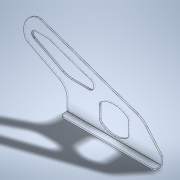
# Autodesk Inventor part: 0 零件
Saved by Autodesk Inventor 2020 (Build 240168000, 168)
## iProperties
Created: 2020-11-03
Part Number: 0 零件
Material: 不鏽鋼
Document SubType Name: Sheet Metal
Designer: p2013
Density: 8 g/cm^3
Appearance: 半拋光
Flat Pattern Width: 10.0917 cm
Flat Pattern Length: 19 cm
Flat Pattern Area: 191.742 cm^2
Sheet Metal Rule: 預設 mm (_M)
Sheet Metal Width: 100.92 mm
Sheet Metal Length: 190.00 mm
Sheet Metal Area: 19174.16 mm^2
Author: p2013
Autodesk Inventor part; units mm, degrees
ref_plane "YZ Plane" through (0, 0, 0) normal (1, 0, 0) x (0, 1, 0)
ref_plane "XZ Plane" through (0, 0, 0) normal (0, 1, 0) x (-1, 0, 0)
ref_plane "XY Plane" through (0, 0, 0) normal (0, 0, 1) x (1, 0, 0)
sketch "草圖1" plane through (0, 0, 0) normal (0, 0, 1) x (1, 0, 0)
  line L0 (0, 0) -> (-40.5681, 0) construction
  line L1 (0, 0) -> (0, 42.2738) construction
  line L2 (-65, 18.7) -> (-19.3972, 18.7) construction
  line L3 (65, 18.7) -> (65, 3.5)
  line L4 (61.5, 0) -> (-61.5, 0)
  line L5 (-65, 3.5) -> (-65, 18.7)
  line L6 (-85.1195, 8.7) -> (78.7394, 8.7)
  arc A0 (-65, 3.5) -> (-61.5, 0) centre (-61.5, 3.5) ccw
  arc A1 (61.5, 0) -> (65, 3.5) centre (61.5, 3.5) ccw
  arc A2 (-18, 17.0607) -> (18, 17.0607) centre (0, 41.0607) ccw
  line L7 (-20, 18.7) -> (20, 18.7) construction
  line L8 (19.3972, 18.7) -> (65, 18.7) construction
  line L9 (-65, 18.7) -> (-65, 23.7)
  line L10 (-75.8518, 41.4851) -> (-119.064, 63.7122)
  line L11 (-101.9165, 99.0537) -> (30.9171, 52.7442)
  line L12 (44.0225, 43.7) -> (65, 18.7)
  arc A3 (44.0225, 43.7) -> (30.9171, 52.7442) centre (21.0412, 24.4164) ccw
  arc A4 (-65, 23.7) -> (-75.8518, 41.4851) centre (-85, 23.7) ccw
  arc A5 (-108.162, 99.165) -> (-124.1228, 69.9202) centre (-101.1042, 76.3353) ccw
  line L13 (-104.5691, 99.9785) -> (-122.3532, 65.4041) construction
  line L14 (-92.566, 80.8091) -> (-108.8509, 80.8091)
  arc A6 (-89.2737, 80.2516) -> (-92.566, 80.8091) centre (-92.566, 70.8091) ccw
  line L15 (-32.7123, 60.5304) -> (-89.2737, 80.2516)
  arc A7 (-108.8509, 80.8091) -> (-110.452, 74.1968) centre (-108.8509, 77.3091) ccw
  line L16 (-110.452, 74.1968) -> (-70.3705, 53.5781)
  arc A8 (-70.3705, 53.5781) -> (-58.9345, 50.8091) centre (-58.9345, 75.8091) ccw
  line L17 (-58.9345, 50.8091) -> (-34.3585, 50.8091)
  arc A9 (-34.3585, 50.8091) -> (-32.7123, 60.5304) centre (-34.3585, 55.8091) ccw
  arc A10 (-88.7798, 81.668) -> (-92.566, 82.3091) centre (-92.566, 70.8091) ccw
  line L18 (-92.566, 82.3091) -> (-108.8509, 82.3091)
  arc A11 (-108.8509, 82.3091) -> (-111.1381, 72.8629) centre (-108.8509, 77.3091) ccw
  line L19 (-111.1381, 72.8629) -> (-71.0567, 52.2443)
  arc A12 (-71.0567, 52.2443) -> (-58.9345, 49.3091) centre (-58.9345, 75.8091) ccw
  line L20 (-58.9345, 49.3091) -> (-34.3585, 49.3091)
  arc A13 (-34.3585, 49.3091) -> (-32.2185, 61.9468) centre (-34.3585, 55.8091) ccw
  line L21 (-32.2185, 61.9468) -> (-88.7798, 81.668)
  arc A14 (-101.9165, 99.0537) -> (-108.162, 99.165) centre (-105.2084, 89.6111) ccw
  arc A15 (-124.1228, 69.9202) -> (-119.064, 63.7122) centre (-114.4899, 72.6048) ccw
  arc A16 (18, 42.7) -> (-18, 42.7) centre (0, 18.7) ccw
  line L22 (-20, 38.7) -> (-20, 21.0607)
  line L23 (20, 38.7) -> (20, 21.0607)
  arc A17 (20, 38.7) -> (18, 42.7) centre (15, 38.7) ccw
  arc A18 (18, 17.0607) -> (20, 21.0607) centre (15, 21.0607) ccw
  arc A19 (-20, 21.0607) -> (-18, 17.0607) centre (-15, 21.0607) ccw
  arc A20 (-18, 42.7) -> (-20, 38.7) centre (-15, 38.7) ccw
  point P0 (0, 0)
  point P1 (20, 41.0607)
  point P2 (-20, 41.0607)
  dimension "d0" = 130
  dimension "d1" = 3.5
  dimension "d2" = 8.7
  dimension "d3" = 10
  dimension "d9" = 2.3607
  dimension "d11" = 30
  dimension "d12" = 117.22
  dimension "d13" = 20
  dimension "d14" = 8
  dimension "d15" = 5
  dimension "d16" = 23.8958
  dimension "d17" = 50
  dimension "d18" = 25
  dimension "d19" = 1.5
  dimension "d20" = 60
  dimension "d21" = 10
  dimension "d22" = 10
  dimension "d23" = 30
  dimension "d24" = 30
  dimension "d25" = 5
  dimension "d26" = 40
  constraints: 49 point on circle, 48 end point, 21 centre point, 20 tangent, 11 point on line, 7 horizontal, 6 equal radius, 6 perpendicular, 4 parallel, 3 midpoint, 2 vertical, 1 coincident, 1 vertical alignment, 27 other
  measures "d0" distance between parallel lines of L3 L5
  measures "d1" radius of A0
  measures "d2" distance between parallel lines of L6 L4
  measures "d3" distance between parallel lines of L6 L2
  measures "d9" distance edge to line of A2 L6
  measures "d11" radius of A3
  measures "d12" angle of L9 L10
  measures "d13" radius of A4
  measures "d14" angle of L10 L11
  measures "d15" distance of L2.start L9.end
  measures "d16" radius of A5
  measures "d17" angle of L8 L12
  measures "d18" vertical distance of L12.start L3.start
  measures "d19" distance between parallel lines of L19 L16
  measures "d21" radius of A14
  measures "d22" distance edge to line of A5 L13
  measures "d23" radius of A16
  measures "d24" distance edge to line of A16 L7
  measures "d25" radius of A17
  measures "d26" distance between parallel lines of L23 L22
extrude "擠出1" add sketch "草圖1" against normal blind 2 contours L3 L6 L5 L9 A4 L10 A15 A5 A14 L11 A3 L12 | L3 A1 L4 A0 L5 L6
bend part "折彎零件1" radius 0.4 angle 85 line through (-85.1195, 8.7, 0) along (1, 0, 0) centre toward (0, 0, 1) moving side (0, -1, 0) both sides no
equation "\"折彎半徑\" = 厚度"
equation "\"折彎離隙寬度\" = 厚度"
equation "\"折彎離隙深度\" = 0.5 * 厚度"
equation "\"轉角離隙大小\" = 4 * 厚度"
equation "\"最小剩餘\" = 2 * 厚度"
equation "\"轉移半徑\" = 折彎半徑"
equation "\"Jacobi半徑大小\" = 折彎半徑"
equation "\"間隙大小\" = 厚度"
equation "\"厚度\" = 2"
